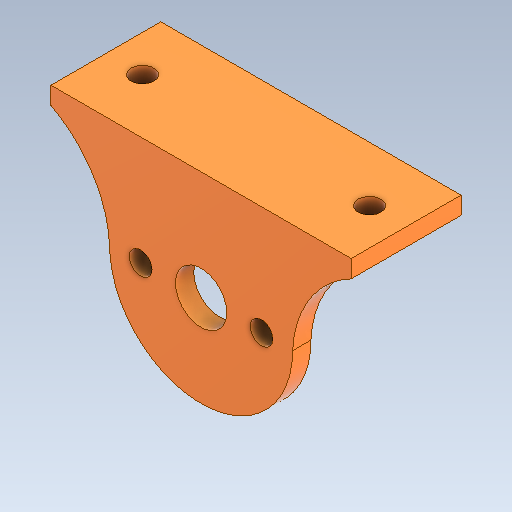
# Autodesk Inventor part: main_motor_mount
Saved by Autodesk Inventor 2020.3 (Build 243373000, 373)
## iProperties
Created: 2020-06-20
Part Number: main_motor_mount
Material: Prusament PETG
Document SubType Name: Modeling
Designer: Devin
Density: 1.541 g/cm^3
Appearance: Polycarbonate - Clear(1)
Mass: 4.39518 g
Surface Area: 28.2224 cm^2
Volume: 2.85216 cm^3
Author: Devin
Autodesk Inventor part; units mm, degrees
ref_plane "YZ Plane" through (0, 0, 0) normal (1, 0, 0) x (0, 1, 0)
ref_plane "XZ Plane" through (0, 0, 0) normal (0, 1, 0) x (-1, 0, 0)
ref_plane "XY Plane" through (0, 0, 0) normal (0, 0, 1) x (1, 0, 0)
sketch "Sketch1" plane through (0, 0, 0) normal (0, 0, 1) x (1, 0, 0)
  circle A0 centre (0, 0) radius 3.5
  circle A1 centre (8.25, 0) radius 1.55
  circle A2 centre (-8.25, 0) radius 1.55
  line L0 (0, 0) -> (0, 12.5)
  line L1 (0, 12.5) -> (12.5, 12.5)
  line L2 (12.5, 0) -> (12.5, 12.5)
  line L3 (0, 12.5) -> (-12.5, 12.5)
  line L4 (-12.5, 12.5) -> (-12.5, 0)
  arc A3 (-12.5, 0) -> (12.5, 0) centre (0, 0) ccw
  dimension "d0" = 7
  dimension "d4" = 3.1
  dimension "d5" = 3.1
  dimension "d9" = 12.5
  dimension "d10" = 12.5
  constraints: 10 end point, 4 centre point, 3 perpendicular, 2 coincident, 2 point on circle, 1 tangent, 1 vertical
  measures "d0" diameter of A0
  measures "d4" diameter of A1
  measures "d5" diameter of A2
  measures "d9" distance of L0.start L0.end
  measures "d10" distance of L0.end L3.end
extrude "Extrusion1" add sketch "Sketch1" along normal blind 2.5
sketch "Sketch2" plane through (0, 0, 2.5) normal (0, 0, 1) x (1, 0, 0)
  line L0 (-12.5, 12.5) -> (-12.5, 0) projected
  line L1 (12.5, 0) -> (12.5, 12.5) projected
  line L2 (-12.5, 12.5) -> (12.5, 12.5)
  line L3 (12.5, 14.9) -> (-12.5, 14.9)
  line L4 (-12.5, 12.5) -> (-20.5, 12.5)
  line L5 (-20.5, 12.5) -> (-20.5, 14.9)
  line L6 (-20.5, 14.9) -> (-12.5, 14.9)
  line L7 (12.5, 12.5) -> (20.5, 12.5)
  line L8 (20.5, 12.5) -> (20.5, 14.9)
  line L9 (20.5, 14.9) -> (12.5, 14.9)
  point P0 (0, 0)
  dimension "d14" = 8
  dimension "d15" = 2.4
  dimension "d17" = 2.4
  constraints: 16 end point, 3 parallel, 2 horizontal, 2 perpendicular, 1 point on line
  measures "d14" distance of L0.start L4.end
  measures "d15" distance of L4.end L5.end
  measures "d17" distance of L8.end L7.end
extrude "Extrusion2" add sketch "Sketch2" against normal blind 15
sketch "Sketch3" plane through (0, 0, 2.5) normal (0, 0, 1) x (1, 0, 0)
  arc A0 (-12.5, 0) -> (12.5, 0) centre (0, 0) ccw projected
  line L0 (20.5, 12.5) -> (-20.5, 12.5) projected
  line L1 (12.5, 12.5) -> (-12.5, 12.5) projected
  arc A1 (-12.5, 0) -> (-20.5, 12.5) centre (-27.4799, -0.7771) ccw
  arc A2 (20.5, 12.5) -> (12.5, 0) centre (27.4799, -0.7771) ccw
  line L2 (-20.5, 12.5) -> (-12.5, 12.5)
  line L3 (-12.5, 12.5) -> (-12.5, 0) projected
  line L4 (-12.5, 0) -> (-12.5, 12.5)
  line L5 (12.5, 0) -> (12.5, 12.5) projected
  line L6 (12.5, 0) -> (12.5, 12.5)
  line L7 (12.5, 12.5) -> (20.5, 12.5)
  dimension "d20" = 15
  dimension "d21" = 15
  constraints: 8 end point, 4 point on circle, 2 centre point, 2 collinear, 2 perpendicular
  measures "d20" radius of A1
  measures "d21" radius of A2
extrude "Extrusion3" add sketch "Sketch3" against normal up to surface (2.5 mm away) contours A1 L0 L3 | L5 L0 A2
sketch "Sketch4" plane through (-20.5, 14.9, 2.5) normal (0, 1, 0) x (1, 0, 0)
  line L0 (41, 15) -> (0, 15) projected
  line L1 (0, 0) -> (0, 15) projected
  line L2 (41, 0) -> (41, 15) projected
  line L3 (41, 7.5) -> (36, 7.5)
  circle A0 centre (5, 7.5) radius 1.55
  circle A1 centre (36, 7.5) radius 1.55
  point P0 (20.5, 2.5)
  dimension "d27" = 3.1
  dimension "d28" = 3.1
  constraints: 2 centre point, 2 end point, 1 coincident, 1 midpoint
  measures "d27" diameter of A0
  measures "d28" diameter of A1
extrude "Extrusion4" cut sketch "Sketch4" against normal blind 10
body "Solid1"
